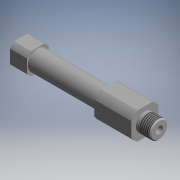
# Autodesk Inventor part: 10-CJ2B10-15RZ(1_0)_BODY
Saved by Autodesk Inventor 2017.3 (Build 213256000, 256)
## iProperties
Part Number: 10-CJ2B10-15RZ(1_0)_BODY
Material: Generic
Catalog Web Link: www.cadenas.de
Description: 10/11-CJ2-Z BODY-Air Cylinder/Standard: Double Acting Single Rod/Clean Series
Vendor: SMC
Document SubType Name: Modeling
Designer: partserver
Manufacturer: SMC
Mass: 7.66763 g
Surface Area: 48.4478 cm^2
Volume: 7.66763 cm^3
Density: 1 g/cm^3
Appearance: PSOLRGB-192-192-192
Category: PARTsolutions
Company: SMC
Title: 10-CJ2B10-15RZ_BODY
Author: Cadenas PARTsolutions
Comments: Air Cylinder/Standard: Double Acting Single Rod/Clean Series
PSOL_IDENT_0: {$CADENAS_DATA\23d-libs\smc_jp\actuator\standard_air_cylinder\cj2\10_cj2_z\parts\10_cj2_z_body.prj},
PSOL_IDENT_1: 263 {VTYP=3D},{NB=10-CJ2B10-15RZ(1_0)_BODY},{LINA=10-CJ2B10-15RZ_BODY},{NN=10/11-CJ2-Z BODY},{DATE=2
PSOL_IDENT_2: 9.10.2021 06:22:37},{GEOMDATE=10.07.2020 03:17:49},{VERSION=},{LINEID=370},{WBVAR=TYPE,AUTOSWITCH,NU
PSOL_IDENT_3: MBER,CUSHION,STOP,STROKE,PORT,MOUNTING,THREAD},{WBNUMERIC=STROKE}  {NB=10-CJ2B10-15RZ(1_0)_BODY},{LI
PSOL_IDENT_4: NA=10-CJ2B10-15RZ_BODY},{KT=DUMMY},{ORDER=10-CJ2B10-15RZ},{TYPE=10},{BORE=10},{MOUNT=(B) Basic},{AUT
PSOL_IDENT_5: OSWITCH=},{NUMBER=},{CUSHION=},{CUSHIONX= '', '(-) Rubber cushion', 'A', '(A) Air cushion' },{MOUNTX=
PSOL_IDENT_6: B},{STOP=1},{STROKE=15},{SMAX=150},{PORT=R},{MOUNTING=},{THREAD=0},{B=15.0},{B1X1=15.0},{B2=15.000},
PSOL_IDENT_7: {C=17.000},{C1X1=17.0},{C2=17.000},{CD=0.0},{U=0},{CX=0.0},{CZ=0},{CZ1X1=0.0},{D=4},{F=8},{GA=8.0},{
PSOL_IDENT_8: GA1X1=8.0},{GA2=7.500},{GB=5.0},{GB1X1=5.0},{GB2=6.500},{H=28},{NA=20.5},{NA1X1=20.5},{NA2=29.500},{
PSOL_IDENT_9: NB1=9.5},{NB1X1=9.5},{NB2=20.000},{NDH8=8 0/-0.022},{NDH81=8},{NN=M10x1.0},{NNN=M10x1.0},{NN1=10},{N
PSOL_IDENT_10: N2=1.0},{R=0},{S=54.000},{S1X1=54.0},{S2X2=73.5},{WA=14.5},{WB=13.5},{WW=4.5},{MOUNTINGX='','(-) Non
PSOL_IDENT_11: e','-B','(B) Band mounting'},{PORTX='', '(-) Perpendicular', 'R', '(R) In-line'},{SWX=4.5},{SW1=6.00
PSOL_IDENT_12: 0},{SW2=2.000},{SW3=2.500},{SW4=1.500},{SW5=4.500},{SW6=0.500},{SW7=3.000},{SW8=3.500},{SW9=0.500},{
PSOL_IDENT_13: SW=4.5},{SWSINX= '','N/A' },{NENN=10-CJ2B10},{X1=6.000},{X2=7.750},{Y1=2.300},{Y2=6.750},{X=6},{Y=2.
PSOL_IDENT_14: 3}
NB: 10-CJ2B10-15RZ(1_0)_BODY
NN: M10x1.0
NT: Air Cylinder/Standard: Double Acting Single Rod/Clean Series
NBSYN: $ORDER.($STOP._$THREAD.)_BODY
LINA: 10-CJ2B10-15RZ_BODY
CATALOG: SMC (JP
ROWDESC: 10-CJ2B10
TYPE: (10) Relief type
BORE: 10
MOUNT: (B) Basic
AUTOSWITCH: (-) Without autoswitch
NUMBER: N/A
CUSHION: (-) Rubber cushion
STOP: Manufacturable stroke
STROKE: 15
SMAX: 150
PORT: (R) In-line
MOUNTING: (-) None
THREAD: on
B: 15
B1X1: 15
B2: 15
C: 17
C1X1: 17
C2: 17
CD: 0
U: 0
CX: 0
CZ: 0
CZ1X1: 0
D: 4
F: 8
GA: 8
GA1X1: 8
GA2: 7.5
GB: 5
GB1X1: 5
GB2: 6.5
H: 28
NA: 20.5
NA1X1: 20.5
NA2: 29.5
NB1: 9.5
NB1X1: 9.5
NB2: 20
NDH8: 8 0/-0.022
NDH81: 8
NNN: M10x1.0
NN1: 10
NN2: 1
R: 0
S: 54
S1X1: 54
S2X2: 73.5
WA: 14.5
WB: 13.5
WW: 4.5
SW1: 6
SW2: 2
SW3: 2.5
SW4: 1.5
SW5: 4.5
SW6: 0.5
SW7: 3
SW8: 3.5
SW9: 0.5
X1: 6
X2: 7.75
Y1: 2.3
Y2: 6.75
SUPPLIER: SMC
ARTICLENO: 10-CJ2B10-15RZ(1_0)_BODY
BOMINFO: 10-CJ2B10-15RZ_BODY
CREATOR: CADENAS GmbH
Autodesk Inventor part; units mm, degrees
sketch "Sketch_8" plane through (0, 0, 0) normal (0, 0, 1) x (1, 0, 0)
  line L0 (0, 0) -> (-8, 0)
  line L1 (-8, 0) -> (-8, 4.3865)
  line L2 (-8, 4.3865) -> (-7.3865, 5)
  line L3 (-7.3865, 5) -> (0, 5)
  line L4 (0, 5) -> (0, 0)
  line L5 (0, 0) -> (-8, 0)
  constraints: 12 end point
revolve "Revolution1" add sketch "Sketch_8" angle 360 about axis through (0, 0, 0) along (1, 0, 0)
thread "Thread1" size "M10x1" class "6g" standard "ISO Metric profile" length 5.8865
sketch "Sketch_9" plane through (0, 0, 0) normal (1, 0, 0) x (0, 0, -1)
  line L0 (-7.5, 4) -> (-7.5, -4)
  arc A0 (-7.5, -4) -> (-4, -7.5) centre (0, 0) ccw
  line L1 (-4, -7.5) -> (4, -7.5)
  arc A1 (4, -7.5) -> (7.5, -4) centre (0, 0) ccw
  line L2 (7.5, -4) -> (7.5, 4)
  arc A2 (7.5, 4) -> (4, 7.5) centre (0, 0) ccw
  line L3 (4, 7.5) -> (-4, 7.5)
  arc A3 (-4, 7.5) -> (-7.5, 4) centre (0, 0) ccw
  constraints: 8 end point, 8 point on circle, 4 centre point
extrude "Extrusion1" add sketch "Sketch_9" along normal blind 20.5
sketch "Sketch_6" plane through (20.5, 0, 0) normal (1, 0, 0) x (0, 0, -1)
  circle A0 centre (0, 0) radius 5.5
  constraints: 1 centre point
extrude "Extrusion2" add sketch "Sketch_6" along normal blind 39
sketch "Sketch_10" plane through (59.5, 0, 0) normal (1, 0, 0) x (0, 0, -1)
  line L0 (-6, 3.6056) -> (-6, -3.6056)
  arc A0 (-6, -3.6056) -> (-3.6056, -6) centre (0, 0) ccw
  line L1 (-3.6056, -6) -> (3.6056, -6)
  arc A1 (3.6056, -6) -> (6, -3.6056) centre (0, 0) ccw
  line L2 (6, -3.6056) -> (6, 3.6056)
  arc A2 (6, 3.6056) -> (3.6056, 6) centre (0, 0) ccw
  line L3 (3.6056, 6) -> (-3.6056, 6)
  arc A3 (-3.6056, 6) -> (-6, 3.6056) centre (0, 0) ccw
  constraints: 8 end point, 8 point on circle, 4 centre point
extrude "Extrusion3" add sketch "Sketch_10" along normal blind 9.5
sketch "Sketch7" plane through (0, 0, 0) normal (0, 0, 1) x (1, 0, 0)
  line L0 (5, 7.5) -> (5, 2.5)
  line L1 (5, 1.3066) -> (2.933, 2.5)
  line L2 (2.933, 2.5) -> (2.933, 7.067)
  line L3 (2.933, 7.067) -> (2.5, 7.5)
  line L4 (2.5, 7.5) -> (5, 7.5)
  line L5 (5, 7.5) -> (5, 1.3066)
  constraints: 12 end point
revolve "Revolution2" cut sketch "Sketch7" angle 360 about axis through (5, 7.5, 0) along (0, 1, 0)
thread "Thread2" size "M5x0.8" class "6H" standard "ISO Metric profile" full length
sketch "Sketch_28" plane through (0, 0, 0) normal (0, 0, 1) x (1, 0, 0)
  line L0 (16, 7.5) -> (16, 2.5)
  line L1 (16, 1.3066) -> (13.933, 2.5)
  line L2 (13.933, 2.5) -> (13.933, 7.067)
  line L3 (13.933, 7.067) -> (13.5, 7.5)
  line L4 (13.5, 7.5) -> (16, 7.5)
  line L5 (16, 7.5) -> (16, 1.3066)
  constraints: 12 end point
revolve "Revolution3" cut sketch "Sketch_28" angle 360 about axis through (16, 7.5, 0) along (0, 1, 0)
thread "Thread3" size "M5x0.8" class "6H" standard "ISO Metric profile" full length
sketch "Sketch8" plane through (0, 0, 0) normal (0, 0, 1) x (1, 0, 0)
  line L0 (69, 0) -> (64, 0)
  line L1 (62.8066, 0) -> (64, 2.067)
  line L2 (64, 2.067) -> (68.567, 2.067)
  line L3 (68.567, 2.067) -> (69, 2.5)
  line L4 (69, 2.5) -> (69, 0)
  line L5 (69, 0) -> (62.8066, 0)
  constraints: 12 end point
revolve "Revolution4" cut sketch "Sketch8" angle 360 about axis through (69, 0, 0) along (1, 0, 0)
thread "Thread4" size "M5x0.8" class "6H" standard "ISO Metric profile" full length
sketch "Sketch_16" plane through (0, 0, 0) normal (0, 0, 1) x (1, 0, 0)
  line L0 (40.5, 0) -> (-8, 0)
  line L1 (-8, 0) -> (-8, 2)
  line L2 (-8, 2) -> (20.5, 2)
  line L3 (20.5, 2) -> (20.5, 5)
  line L4 (20.5, 5) -> (40.5, 5)
  line L5 (40.5, 5) -> (40.5, 0)
  line L6 (40.5, 0) -> (-8, 0)
  constraints: 14 end point
revolve "Revolution5" cut sketch "Sketch_16" angle 360 about axis through (40.5, 0, 0) along (1, 0, 0)
ref_plane "BODY_N_XY" through (77, 0, 0) normal (0, 0, -1) x (1, 0, 0)
ref_plane "BODY_N_YZ" through (77, 0, 0) normal (1, 0, 0) x (0, -1, 0)
ref_plane "BODY_N_ZX" through (77, 0, 0) normal (0, -1, 0) x (0, 0, -1)
ref_plane "NUT2_XY" through (69, 0, 0) normal (1, 0, 0) x (0, 0, -1)
ref_plane "NUT2_YZ" through (69, 0, 0) normal (0, 0, -1) x (0, 1, 0)
ref_plane "NUT2_ZX" through (69, 0, 0) normal (0, 1, 0) x (1, 0, 0)
ref_plane "SW1_XY" through (25, 0, 0) normal (1, 0, 0) x (0, 0, -1)
ref_plane "SW1_YZ" through (25, 0, 0) normal (0, 0, -1) x (0, 1, 0)
ref_plane "SW1_ZX" through (25, 0, 0) normal (0, 1, 0) x (1, 0, 0)
ref_plane "SW2_XY" through (55, 0, 0) normal (-1, 0, 0) x (0, 0, -1)
ref_plane "SW2_YZ" through (55, 0, 0) normal (0, 0, -1) x (0, -1, 0)
ref_plane "SW2_ZX" through (55, 0, 0) normal (0, -1, 0) x (-1, 0, 0)
ref_plane "SW_R1_XY" through (25, -12.5, 0) normal (1, 0, 0) x (0, 0, -1)
ref_plane "SW_R1_YZ" through (25, -12.5, 0) normal (0, 0, -1) x (0, 1, 0)
ref_plane "SW_R1_ZX" through (25, -12.5, 0) normal (0, 1, 0) x (1, 0, 0)
ref_plane "SW_R2_XY" through (55, -12.5, 0) normal (-1, 0, 0) x (0, 0, -1)
ref_plane "SW_R2_YZ" through (55, -12.5, 0) normal (0, 0, -1) x (0, -1, 0)
ref_plane "SW_R2_ZX" through (55, -12.5, 0) normal (0, -1, 0) x (-1, 0, 0)
ref_plane "body_XY" through (0, 0, 0) normal (1, 0, 0) x (0, 0, -1)
ref_plane "body_YZ" through (0, 0, 0) normal (0, 0, -1) x (0, 1, 0)
ref_plane "body_ZX" through (0, 0, 0) normal (0, 1, 0) x (1, 0, 0)
body "Solid1"
